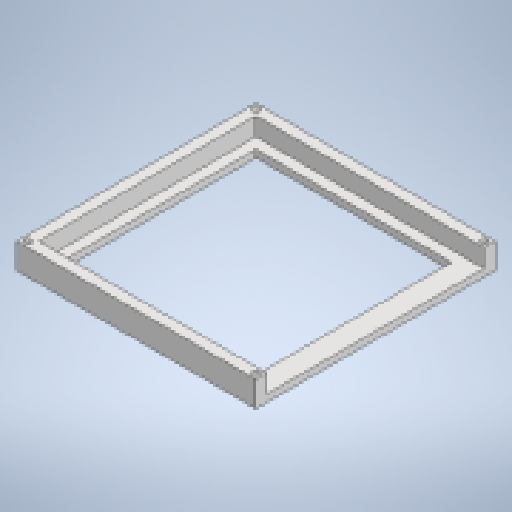
# Autodesk Inventor part: Disco_inferior
Saved by Autodesk Inventor 2024 (Build 280153000, 153)
## iProperties
Created: 2025-02-27
Part Number: Disco_inferior
Material: Genérico
Document SubType Name: Modeling
Designer: sergi
Density: 1 g/cm^3
Appearance: Valor por defecto
Author: sergi
Autodesk Inventor part; units mm, degrees
ref_plane "YZ Plane" through (0, 0, 0) normal (1, 0, 0) x (0, 1, 0)
ref_plane "XZ Plane" through (0, 0, 0) normal (0, 1, 0) x (-1, 0, 0)
ref_plane "XY Plane" through (0, 0, 0) normal (0, 0, 1) x (1, 0, 0)
sketch "Boceto1" plane through (0, 0, 0) normal (0, 1, 0) x (-1, 0, 0)
  line L0 (0, 0) -> (60, 0)
  line L1 (60, 0) -> (60, 60)
  line L2 (60, 60) -> (0, 60)
  line L3 (0, 60) -> (0, 0)
  line L4 (3, 57) -> (57, 57)
  line L5 (57, 57) -> (57, 3)
  line L6 (57, 3) -> (3, 3)
  line L7 (3, 3) -> (3, 57)
  line L8 (-3, 63) -> (63, 63)
  line L9 (63, 63) -> (63, -3)
  line L10 (63, -3) -> (-3, -3)
  line L11 (-3, -3) -> (-3, 63)
  dimension "d0" = 60
  dimension "d1" = 60
  dimension "d3" = 3
  dimension "d13" = 3
  constraints: 24 end point, 6 parallel, 3 perpendicular, 1 horizontal, 6 other
  measures "d0" distance of L2.end L1.end
  measures "d1" distance of L0.end L1.end
  measures "d3" distance between parallel lines of L2 L8
  measures "d13" distance between parallel lines of L2 L4
extrude "Extrusión1" add sketch "Boceto1" along normal blind 6 contours L8 L9 L10 L11
sketch "Boceto2" plane through (0, 0, 0) normal (0, -1, 0) x (1, 0, 0)
  line L0 (3, -3) -> (-63, -3) projected
  line L1 (3, 63) -> (3, -3) projected
  line L2 (-63, 63) -> (3, 63) projected
  line L3 (-63, -3) -> (-63, 63) projected
  line L4 (0, 0) -> (0, 60) projected
  line L5 (-60, 0) -> (0, 0) projected
  line L6 (-60, 60) -> (-60, 0) projected
  line L7 (0, 60) -> (-60, 60) projected
extrude "Extrusión2" add sketch "Boceto2" along normal blind 2 contours L0 L3 L2 L1 | L5 L6 L7 L4
sketch "Boceto3" plane through (0, 6, 0) normal (0, 1, 0) x (1, 0, 0)
  line L0 (0, 0) -> (0, -60) projected
  line L1 (0, -60) -> (3, -60)
  line L2 (3, -60) -> (3, 0)
  line L3 (3, 0) -> (0, 0)
  line L4 (0, 0) -> (0, -60)
  constraints: 8 end point, 2 parallel, 1 horizontal, 1 perpendicular
extrude "Extrusión3" cut sketch "Boceto3" against normal up to surface (6 mm away)
sketch "Boceto4" plane through (0, 0, 0) normal (0, 1, 0) x (1, 0, 0)
  line L0 (-60, 0) -> (3, 0) projected
  line L1 (-60, -60) -> (-60, 0) projected
  line L2 (-60, -60) -> (3, -60) projected
  line L3 (3, 0) -> (3, -60) projected
  line L4 (3, -60) -> (0, -60)
  line L5 (0, -60) -> (0, 0)
  line L6 (0, -57) -> (0, -3)
  line L7 (0, -3) -> (-57, -3)
  line L8 (-57, -3) -> (-57, -57)
  line L9 (-57, -57) -> (0, -57)
  line L10 (-3, 0) -> (-3, -63)
  line L11 (-3, -63) -> (3, -63)
  point P0 (-3, -57)
  point P1 (-3, -3)
  dimension "d28" = 3
  constraints: 16 end point, 2 point on line, 1 perpendicular, 4 other
  measures "d28" distance of L2.end L4.end
extrude "Extrusión4" cut sketch "Boceto4" against normal blind 10 contours L10 L9 L8 L7
fillet "Empalme1" radius 10 4 edges at (-3, -1, 57) (-3, -1, 3) (-57, -1, 3) (-57, -1, 57)
